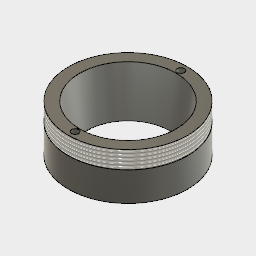
B-table and Collet v2 (Autodesk Fusion 360 archive; units mm, degrees)
design "Collet Bottom Taper"
Autodesk Fusion 360 part; units mm, degrees
sketch "Sketch1" plane through (0, 0, 0) normal (0, 0, 1) x (1, 0, 0)
  line L0 (-18.15, 0) -> (-25.95, 0)
  line L1 (-25.95, 0) -> (-25.95, 12.7)
  line L2 (-25.95, 12.7) -> (-26.375, 12.7)
  line L3 (-26.375, 12.7) -> (-26.375, 20.32)
  line L4 (-26.375, 20.32) -> (-21.0058, 20.32)
  line L5 (-21.0058, 20.32) -> (-18.15, 0)
  dimension "d1" = 25.95
  dimension "d2" = 26.375
  dimension "d3" = 12.7
  dimension "d4" = 7.62
  dimension "d5" = 98
  dimension "d6" = 7.8
  dimension "d7" = 20.32
  measures "d1" distance of origin L1
  measures "d2" distance of origin L3
  measures "d3" distance of L0.end L1.end
  measures "d4" distance of L2.end L3.end
  measures "d5" angle of L0 L5
  measures "d6" distance of L0.end L0.start
  measures "d7" distance of origin L4.end
sketch "Sketch2" plane through (0, 0, 0) normal (0, 0, 1) x (1, 0, 0)
  line L0 (-18.15, 0) -> (-25.95, 0)
  line L1 (0, 0) -> (0, 22) construction
revolve "Revolve1" add sketch "Sketch1" angle 360 about axis through (0, 0, 0) along (0, 1, 0)
thread "Thread1" "ISO Metric profile 52.0 M52x1.5 6g" major diameter 51.85 minor diameter 50.1269 pitch 1.5 angle 60 resizes the face on face at (-26.3422, 15.24, -1.3147)
sketch "Sketch3" plane through (0, 20.32, 0) normal (0, 1, 0) x (-1, 0, 0)
  circle A0 centre (0, 0) radius 25.925
  circle A1 centre (0, 0) radius 21.0058
  point P0 (0, -23)
  point P1 (0, 23)
  dimension "d9" = 46
  dimension "d10" = 23
  measures "d9" distance of P0 P1
  measures "d10" distance of A0.centre P0
hole "Hole1" at (0, 20.32, -23) at (0, 20.32, 23) direction (0, -1, 0) diameter 3.1 depth 13.5 tip angle 118
equation "d1 = ( 51.9 / 2 ) * 1 mm"
equation "d2 = ( 52.75 / 2 ) * 1 mm"

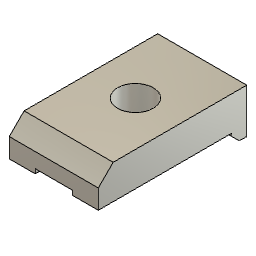
design "CY7 diode clamp"
Autodesk Fusion 360 part; units mm, degrees
sketch "Sketch1" plane through (0, 0, 0) normal (0, 1, 0) x (1, 0, 0)
  line L0 (-3, 4.5) -> (3, 4.5)
  line L1 (3, 4.5) -> (3, -5.5)
  line L2 (3, -5.5) -> (-3, -5.5)
  line L3 (-3, -5.5) -> (-3, 4.5)
  line L4 (-1.25, -5.5) -> (-1.25, -2.5)
  arc A0 (1.25, -2.5) -> (-1.25, -2.5) centre (0, -2.5) ccw
  line L5 (1.25, -2.5) -> (1.25, -5.5)
  line L6 (-3, 3.5) -> (3, 3.5)
  line L7 (0, 0) -> (0, -2.5) construction
  dimension "d2" = 2.5
  dimension "d3" = 3
  dimension "d4" = 1
  dimension "d5" = 10
  dimension "d6" = 2.5
  dimension "d7" = 6
  constraint horizontal L0
  constraint vertical L1
  constraint horizontal L2
  constraint vertical L3
  constraint coincident L2 L4.start
  constraint perpendicular L2 L4
  constraint tangent L4 A0
  constraint coincident L2 L5.end
  constraint tangent A0 L5
  constraint perpendicular L2 L5
  constraint coincident L3 L6.start
  constraint coincident L1 L6.end
  constraint perpendicular L1 L6
  constraint coincident L7.start origin
  constraint vertical L7.start A0.centre
  constraint coincident A0.centre L7.end
  constraint symmetric L1 L3 L7
  measures "d2" distance of L4 L5
  measures "d3" distance of L2 A0.centre
  measures "d4" distance of L0 L6
  measures "d5" distance of L0 L2
  measures "d6" distance of A0.centre L7.start
  measures "d7" distance of L1 L3
extrude "Extrude1" add sketch "Sketch1" along normal blind 3
extrude "Extrude2" cut sketch "Sketch1" along normal blind 0.7 contours L1 L2 L3 L4 A0 L5 L6 | L2 L4 A0 L5
extrude "Extrude3" cut sketch "Sketch1" along normal blind 1 contours L2 L4 A0 L5
hole "Hole1" at (0, 0, 0) direction (0, 1, 0) diameter 2.4 depth 5 tip angle 118
chamfer "Chamfer1" distance 0.5 angle 45 1 edges at (0, 0, -3.5)
chamfer "Chamfer2" distance 1 angle 45 1 edges at (0, 3, 5.5)

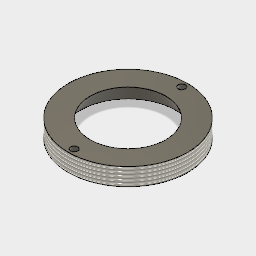
design "Collet Top Taper"
Autodesk Fusion 360 part; units mm, degrees
sketch "Sketch1" plane through (0, 0, 0) normal (0, 0, 1) x (1, 0, 0)
  line L0 (-20.7744, 0) -> (-26.35, 0)
  line L1 (-26.35, 0) -> (-26.35, 7.62)
  line L2 (-26.35, 7.62) -> (-16.375, 7.62)
  line L3 (-16.375, 7.62) -> (-20.7744, 0)
  dimension "d1" = 26.35
  dimension "d2" = 16.375
  dimension "d3" = 60
  dimension "d4" = 7.62
  dimension "d5" = 7.62
  measures "d1" distance of origin L0.end
  measures "d2" distance of origin L2.end
  measures "d3" angle of L0 L3
  measures "d4" distance of L0.end L1.end
  measures "d5" distance of origin L2.end
sketch "Sketch2" plane through (0, 0, 0) normal (0, 0, 1) x (1, 0, 0)
  line L0 (0, 0) -> (0, 1)
  line L1 (0, 1) -> (0, 14) construction
revolve "Revolve1" add sketch "Sketch1" angle 360 about axis through (0, 1, 0) along (0, 1, 0)
thread "Thread1" "ISO Metric profile 52.0 M52x1.5 6g" major diameter 51.85 minor diameter 50.1269 pitch 1.5 angle 60 resizes the face on face at (-26.2191, 2.54, -2.6236)
sketch "Sketch3" plane through (0, 7.62, 0) normal (0, 1, 0) x (-1, 0, 0)
  circle A0 centre (0, 0) radius 25.925
  circle A1 centre (0, 0) radius 16.375
  point P0 (-0.0141, -23.35)
  point P1 (-0.0141, 23.35)
  dimension "d7" = 46.7
  dimension "d8" = 23.35
  measures "d7" distance of P0 P1
  measures "d8" distance of A0.centre P0
hole "Hole1" at (0.0141, 7.62, -23.35) at (0.0141, 7.62, 23.35) direction (0, -1, 0) diameter 3.1 depth 13.5 tip angle 118
equation "d1 = ( 52.7 / 2 ) * 1 mm"
equation "d2 = ( 32.75 / 2 ) * 1 mm"
